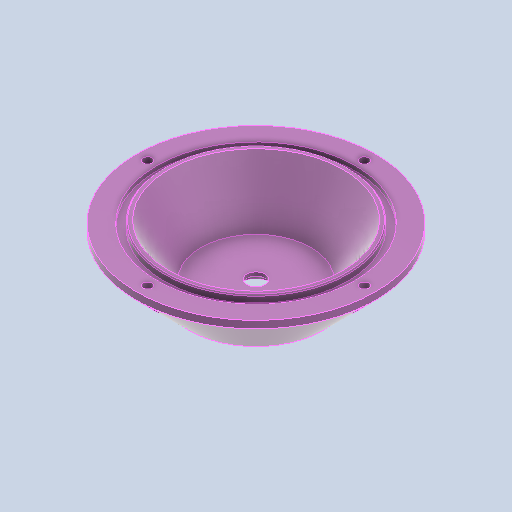
# Autodesk Inventor part: 001
Saved by Autodesk Inventor 2023 (Build 270158000, 158)
## iProperties
Created: 2021-10-30
Part Number: 001
Material: Iron, Cast
Document SubType Name: Modeling
Designer: vinicius.miguel
Density: 7.15 g/cm^3
Appearance: Smooth - Purple
Mass: 117.151 g
Surface Area: 93.5686 cm^2
Volume: 14.9237 cm^3
Author: vinicius.miguel
Autodesk Inventor part; units mm, degrees
ref_plane "YZ Plane" through (0, 0, 0) normal (1, 0, 0) x (0, 1, 0)
ref_plane "XZ Plane" through (0, 0, 0) normal (0, 1, 0) x (-1, 0, 0)
sketch "Sketch1" plane through (0, 0, 0) normal (0, 0, 1) x (1, 0, 0)
  line L0 (4.5, 0) -> (18.2, 0)
  line L1 (32.5, 16.3) -> (27, 16.3)
  line L2 (27, 16.3) -> (27, 15.07)
  line L3 (27, 15.07) -> (25, 15.07)
  line L4 (15, 3) -> (2.5, 3)
  line L5 (2.5, 3) -> (2.5, 2)
  line L6 (0, 0) -> (0, 9.8768)
  line L7 (2.5, 2) -> (4.5, 0)
  line L8 (15, 3) -> (23.7482, 17)
  line L9 (23.7482, 17) -> (25, 17)
  line L10 (25, 17) -> (25, 15.07)
  line L11 (32.5, 14.3) -> (32.5, 16.3)
  line L12 (32.5, 16.3) -> (32.5, 16.3)
  line L13 (18.2, 0) -> (32.5, 14.3)
  point P0 (2.5, 0)
  point P1 (31.0858, 16.3)
  dimension "d0" = 5
  dimension "d1" = 3
  dimension "d11" = 2
  dimension "d12" = 2
  dimension "d20" = 17
  dimension "d23" = 50
  dimension "d24" = 1.23
  dimension "d25" = 2
  dimension "d26" = 30
  dimension "d28" = 65
  dimension "d43" = 32
  dimension "d51" = 16.3
  dimension "d52" = 2
  dimension "d53" = 135
  constraints: 28 end point, 3 perpendicular, 2 horizontal, 2 parallel, 2 point on line, 2 vertical, 1 horizontal alignment
  measures "d0" diameter of L5 L6
  measures "d1" distance of L4.end point (2.5, 0)
  measures "d11" distance of L5.end point (2.5, 0)
  measures "d12" distance of L0.start point (2.5, 0)
  measures "d20" distance from line of L9 L6.start
  measures "d23" diameter of L10 L6
  measures "d24" distance of L1.end L2.end
  measures "d25" distance of L2.end L3.end
  measures "d26" diameter of L4.start L6
  measures "d28" diameter of L1.start L6
  measures "d43" angle of L8 L6
  measures "d51" distance from line of L1 L6.start
  measures "d52" distance of L11.start L1.start
  measures "d53" angle of L13 L0
revolve "Revolution1" add sketch "Sketch1" angle 360 about axis through (0, 0, 0) along (0, 1, 0)
ref_plane "Work Plane1" through (0, 8.3, 0) normal (0, 1, 0) x (1, 0, 0)
sketch "Sketch2" plane through (0, 8.3, 0) normal (0, -1, 0) x (1, 0, 0)
  point P0 (0, 0)
  point P1 (29.5, 0)
  dimension "d38" = 29.5
  measures "d38" distance of point (29.5, 0) point (0, 0)
hole "Hole1" at (29.5, 8.3, 0) direction (0, 1, 0) diameter 2.4 end through all counterbore diameter 4.5 counterbore depth 6 clearance for "Socket Head Cap Screw ISO 4762" size "M2" standard "ISO"
sketch "Sketch4" plane through (29.5, 14.3, 0) normal (0, -1, 0) x (0, 0, -1)
  spline S0 degree 2 poles (2.25, 0) (2.25, -3.8971) (-1.125, -1.9486) (-4.5, 0) (-1.125, 1.9486) (2.25, 3.8971) (2.25, 0) knots 0 0 0 0.333333 0.333333 0.666667 0.666667 1 1 1 weights 1 0.5 1 0.5 1 0.5 1 projected
  line L0 (0, 0) -> (0, 7.8892) construction
  line L1 (2.25, 0) -> (2.25, 7.8892)
  line L2 (-2.25, 7.8892) -> (-2.25, 0)
  arc A0 (-2.25, 0) -> (2.25, 0) centre (0, 0) ccw
  arc A1 (2.25, 7.8892) -> (-2.25, 7.8892) centre (0, 7.8892) ccw
  circle A2 centre (0, 0) radius 2.25 projected
  point P0 (0, -29.5)
  point P1 (0, 3.9446)
  point P2 (-2.25, 0)
  point P3 (2.25, 0)
  constraints: 8 end point, 4 point on circle, 4 tangent, 2 centre point, 1 midpoint, 1 parallel, 1 vertical, 3 other
extrude "Extrusion2" cut sketch "Sketch4" along normal blind 10
pattern_circular "Circular Pattern1" count 4 over 360 about axis through (0, -10, 0) along (0, 1, 0) of "Hole1", "Extrusion2"
chamfer "Chamfer1" distance 0.3 angle 45 1 edges at (-25, 17, 0)
equation "\"d12\" = d11"
body "Solid1"
